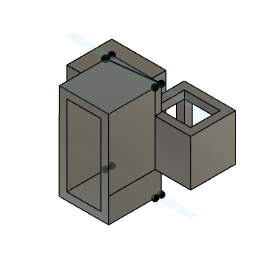
DrzacZaALUFrameKojiDrziKameruZaNogaruStola v4 (Autodesk Fusion 360 design; units mm, degrees)
Autodesk Fusion 360 part; units mm, degrees
sketch "Sketch1" plane through (0, 0, 0) normal (0, 0, 1) x (1, 0, 0)
  line L0 (100, 50) -> (100, 20)
  line L1 (100, 50) -> (150, 50)
  line L2 (120, 20) -> (100, 20)
  line L3 (70, 50) -> (70, 70)
  line L4 (70, 70) -> (150, 70)
  line L5 (100, 50) -> (120, 50)
  line L6 (120, 50) -> (120, 20)
  line L7 (150, 50) -> (150, 70)
  line L8 (150, 50) -> (100, 50)
  line L9 (70, 50) -> (150, 50)
  line L10 (120, 50) -> (150, 50)
  line L11 (100, 50) -> (70, 50)
  line L12 (120, 50) -> (125, 50)
  line L13 (125, 20) -> (125, 50)
  line L14 (125, 20) -> (120, 20)
  line L15 (100, 20) -> (95, 20)
  line L16 (95, 20) -> (95, 50)
  dimension "d1" = 30
  dimension "d2" = 50
  dimension "d3" = 20
  constraint horizontal L9
  constraint coincident L0.start L9
  constraint perpendicular L0 L1
  constraint perpendicular L0 L2
  constraint perpendicular L3 L9
  constraint perpendicular L0 L4
  constraint perpendicular L0 L5
  constraint perpendicular L2 L6
  constraint perpendicular L4 L7
  constraint midpoint L1 L12.end
  constraint perpendicular L8 L13
  constraint perpendicular L6 L14
  constraint perpendicular L0 L15
  constraint coincident L11 L16.end
  measures "d1" distance of L0.start L0.end
  measures "d2" distance of L0.start L1.end
  measures "d3" distance of L0.start L5.end
extrude "Extrude1" add sketch "Sketch1" along normal blind 60
sketch "Sketch2" plane through (0, 20, 0) normal (0, -1, 0) x (1, 0, 0)
  line L0 (95, 0) -> (125, 0)
  line L1 (125, 0) -> (125, 60)
  line L2 (125, 60) -> (95, 60)
  line L3 (95, 60) -> (95, 0)
  line L4 (95, 0) -> (100, 0)
  line L5 (100, 0) -> (100, 55)
  line L6 (100, 55) -> (120, 55)
  line L7 (120, 55) -> (120, 5)
  line L8 (120, 5) -> (100, 5)
  line L9 (-15, -85) -> (-10, -80)
  dimension "d6" = 5
  constraint coincident L0.start L3.end
  constraint perpendicular L3 L4
  constraint perpendicular L4 L5
  constraint perpendicular L5 L6
  constraint perpendicular L6 L7
  constraint coincident L5 L8.end
  constraint perpendicular L5 L8
  measures "d6" distance of L0.start L4.end
extrude "Extrude2" add 1 faces at (105, 63.3333, 60) along direction (0, 0, 1) blind 2
extrude "Extrude3" cut sketch "Sketch2" against normal blind 30 contours L5 L6 L7 L8
extrude "Extrude4" cut 1 faces at (106.6667, 30, 55) along direction (0, 0, 1) blind 2
extrude "Extrude5" add 1 faces at (125, 30, 20.6667) along direction (1, 0, 0) blind 2
extrude "Extrude6" cut 1 faces at (120, 30, 39.6667) along direction (1, 0, 0) blind 2
sketch "Sketch3" plane through (0, 70, 0) normal (0, 1, 0) x (-1, 0, 0)
  line L0 (-150, 0) -> (-70, 0)
  line L1 (-70, 0) -> (-70, 62)
  line L2 (-70, 62) -> (-150, 62)
  line L3 (-150, 62) -> (-150, 0)
  line L4 (-70, 31) -> (-150, 31)
  line L5 (-150, 31) -> (-150, 16)
  line L6 (-150, 31) -> (-150, 46)
  line L7 (-150, 16) -> (-70, 16)
  line L8 (-150, 46) -> (-70, 46)
  dimension "d17" = 15
  dimension "d18" = 15
  constraint midpoint L1 L4.start
  constraint midpoint L3 L4.end
  constraint perpendicular L4 L5
  constraint perpendicular L4 L6
  constraint coincident L1 L7.end
  constraint perpendicular L1 L7
  constraint coincident L1 L8.end
  constraint perpendicular L1 L8
  measures "d17" distance of L4.end L5.end
  measures "d18" distance of L4.end L6.end
extrude "Extrude7" cut sketch "Sketch3" against normal blind 16 contours L0 L1 L3 L7 | L1 L2 L3 L8
sketch "Sketch4" plane through (0, 0, 0) normal (0, 0, -1) x (1, 0, 0)
  line L0 (70, -54) -> (150, -54)
  line L1 (150, -54) -> (150, -50)
  line L2 (150, -50) -> (127, -50)
  line L3 (127, -50) -> (127, -20)
  line L4 (127, -20) -> (95, -20)
  line L5 (95, -20) -> (95, -50)
  line L6 (95, -50) -> (70, -50)
  line L7 (70, -50) -> (70, -54)
  line L8 (127, -50) -> (127, -54)
  line L9 (95, -50) -> (95, -54)
  constraint coincident L2.end L3.start
  constraint coincident L0 L8.end
  constraint perpendicular L0 L8
  constraint coincident L5.end L6.start
  constraint coincident L0 L9.end
  constraint perpendicular L0 L9
sketch "Sketch5" plane through (0, 54, 0) normal (0, 1, 0) x (-1, 0, 0)
  line L0 (-150, 0) -> (-70, 0)
  line L1 (-70, 0) -> (-70, 16)
  line L2 (-70, 16) -> (-150, 16)
  line L3 (-150, 16) -> (-150, 0)
  line L4 (-95, 0) -> (-95, 16)
  line L5 (-126.9826, 0) -> (-126.9826, 16)
  constraint coincident L0 L4.start
  constraint coincident L2 L4.end
  constraint perpendicular L2 L4
  constraint coincident L0 L5.start
  constraint coincident L2 L5.end
  constraint perpendicular L2 L5
extrude "Extrude8" cut sketch "Sketch5" against normal blind 50 contours L0 L2 L3 L5 | L0 L1 L2 L4
sketch "Sketch6" plane through (0, 0, 62) normal (0, 0, 1) x (-1, 0, 0)
  line L0 (-150, -54) -> (-70, -54)
  line L1 (-70, -54) -> (-70, -50)
  line L2 (-70, -50) -> (-95, -50)
  line L3 (-95, -50) -> (-95, -20)
  line L4 (-95, -20) -> (-127, -20)
  line L5 (-127, -20) -> (-127, -50)
  line L6 (-127, -50) -> (-150, -50)
  line L7 (-150, -50) -> (-150, -54)
  line L8 (-127, -50) -> (-127, -54)
  line L9 (-127, -54) -> (-95, -50)
  line L10 (-95, -54) -> (-95, -50)
  constraint coincident L5.end L6.start
  constraint coincident L0 L8.end
  constraint perpendicular L0 L8
  constraint coincident L2.end L3.start
  constraint coincident L0 L10.start
  constraint perpendicular L2 L10
sketch "Sketch7" plane through (0, 54, 0) normal (0, 1, 0) x (-1, 0, 0)
  line L0 (-150, 46) -> (-70, 46)
  line L1 (-70, 46) -> (-70, 62)
  line L2 (-70, 62) -> (-150, 62)
  line L3 (-150, 62) -> (-150, 46)
  line L4 (-95.1201, 62) -> (-95.1201, 46)
  line L5 (-127.0485, 62) -> (-127.0485, 46)
  constraint coincident L2 L4.start
  constraint coincident L0 L4.end
  constraint perpendicular L0 L4
  constraint coincident L2 L5.start
  constraint coincident L0 L5.end
  constraint perpendicular L0 L5
extrude "Extrude9" cut sketch "Sketch7" against normal blind 50 contours L0 L2 L3 L5 | L0 L1 L2 L4
sketch "Sketch8" plane through (0, 0, 0) normal (0, 0, -1) x (1, 0, 0)
extrude "Extrude10" add 1 faces at (96.6667, 70, 36) along direction (0, 1, 0) blind 9
sketch "Sketch9" plane through (0, 0, 62) normal (0, 0, 1) x (1, 0, 0)
sketch "Sketch10" plane through (70, 0, 0) normal (-1, 0, 0) x (0, -1, 0)
  line L0 (-50, 46) -> (-79, 46)
  line L1 (-79, 46) -> (-79, 16)
  line L2 (-79, 16) -> (-50, 16)
  line L3 (-50, 16) -> (-50, 46)
  line L4 (-74, 27.7711) -> (-74, 16)
  line L5 (-74, 27.7711) -> (-74, 46)
  line L6 (-74, 46) -> (-54, 46)
  line L7 (-54, 16) -> (-54, 46)
  line L8 (-54, 16) -> (-54, 21)
  line L9 (-54, 21) -> (-74, 21)
  line L10 (-74, 21) -> (-74, 41)
  line L11 (-74, 41) -> (-54, 41)
  dimension "d28" = 20
  dimension "d29" = 5
  dimension "d30" = 20
  constraint coincident L2 L4.end
  constraint perpendicular L2 L4
  constraint coincident L0 L5.end
  constraint perpendicular L0 L5
  constraint perpendicular L3 L6
  constraint coincident L2 L7.start
  constraint perpendicular L6 L7
  constraint perpendicular L2 L8
  constraint coincident L4 L9.end
  constraint perpendicular L4 L9
  constraint perpendicular L9 L10
  constraint coincident L7 L11.end
  constraint perpendicular L7 L11
  measures "d28" distance of L5.end L6.end
  measures "d29" distance of L7.start L8.end
  measures "d30" distance of L9.end L10.end
extrude "Extrude11" cut sketch "Sketch10" against normal blind 500 contours L4 L5 L7 L9 L10 L11
sketch "Sketch11" plane through (0, 0, 0) normal (0, 1, 0) x (1, 0, 0)
sketch "Sketch12" plane through (0, 79, 0) normal (0, 1, 0) x (-1, 0, 0)
  line L0 (-150, 16) -> (-70, 16)
  line L1 (-70, 16) -> (-70, 46)
  line L2 (-70, 46) -> (-150, 46)
  line L3 (-150, 46) -> (-150, 16)
  line L4 (-94.9405, 16) -> (-94.9405, 46)
  line L5 (-126.875, 16) -> (-126.875, 46)
  line L6 (-94.9405, 16) -> (-99.9405, 16)
  line L7 (-126.875, 16) -> (-121.875, 16)
  line L8 (-99.9405, 16) -> (-105, 16)
  line L9 (-121.875, 16) -> (-116.875, 16)
  line L10 (-105, 16) -> (-105, 46)
  line L11 (-116.875, 16) -> (-116.875, 46)
  dimension "d33" = 5
  dimension "d34" = 5
  dimension "d35" = 5
  constraint coincident L0 L4.start
  constraint coincident L2 L4.end
  constraint perpendicular L2 L4
  constraint coincident L0 L5.start
  constraint coincident L2 L5.end
  constraint perpendicular L2 L5
  constraint perpendicular L4 L6
  constraint perpendicular L5 L7
  constraint coincident L0 L8.end
  constraint parallel L0 L8
  constraint parallel L0 L9
  constraint coincident L2 L10.end
  constraint perpendicular L2 L10
  constraint coincident L2 L11.end
  constraint perpendicular L2 L11
  measures "d33" distance of L4.start L6.end
  measures "d34" distance of L5.start L7.end
  measures "d35" distance of L7.end L9.end
extrude "Extrude12" cut sketch "Sketch12" against normal blind 25 contours L0 L2 L10 L11
sketch "Sketch13" plane through (0, 79, 0) normal (0, 1, 0) x (-1, 0, 0)
  line L0 (-105, 46) -> (-105, 16)
  line L1 (-105, 16) -> (-70, 16)
  line L2 (-70, 16) -> (-70, 46)
  line L3 (-70, 46) -> (-105, 46)
  line L4 (-70, 16) -> (-75, 16)
  line L5 (-70, 16) -> (-70, 21)
  line L6 (-105, 46) -> (-105, 41)
  line L7 (-105, 46) -> (-100, 46)
  line L8 (-105, 16) -> (-105, 17)
  line L9 (-105, 16) -> (-105, 21)
  line L10 (-105, 16) -> (-100, 16)
  line L11 (-70, 46) -> (-75, 46)
  line L12 (-70, 46) -> (-70, 41)
  line L13 (-94, 41) -> (-81, 41)
  line L14 (-75, 25.1667) -> (-75, 36.8333)
  line L15 (-100, 25.1667) -> (-100, 36.8333)
  line L16 (-81, 21) -> (-94, 21)
  line L17 (-75, 36.8333) -> (-82, 31)
  line L18 (-87.5, 26.4167) -> (-94, 21)
  line L19 (-81, 41) -> (-87.5, 35.5833)
  line L20 (-93, 31) -> (-100, 25.1667)
  line L21 (-100, 36.8333) -> (-93, 31)
  line L22 (-87.5, 26.4167) -> (-81, 21)
  line L23 (-75, 25.1667) -> (-82, 31)
  line L24 (-87.5, 35.5833) -> (-94, 41)
  dimension "d38" = 5
  dimension "d39" = 5
  dimension "d40" = 5
  dimension "d41" = 5
  dimension "d42" = 5
  dimension "d43" = 5
  dimension "d44" = 5
  constraint coincident L1.end L2.start
  constraint coincident L0.start L3.end
  constraint coincident L1 L4.end
  constraint perpendicular L2 L4
  constraint perpendicular L4 L5
  constraint perpendicular L3 L6
  constraint perpendicular L6 L7
  constraint coincident L0.end L1.start
  constraint coincident L0 L8.end
  constraint perpendicular L1 L8
  constraint perpendicular L1 L9
  constraint perpendicular L8 L10
  constraint coincident L2.end L3.start
  constraint perpendicular L2 L11
  constraint perpendicular L11 L12
  constraint perpendicular L13 L14
  constraint perpendicular L13 L15
  constraint collinear L17 L18
  constraint coincident L19.end L23
  constraint collinear L19 L20
  constraint coincident L18.start L21
  constraint collinear L21 L22
  constraint collinear L23 L24
  measures "d38" distance of L1.end L5.end
  measures "d39" distance of L0.start L6.end
  measures "d40" distance of L0.start L7.end
  measures "d41" distance of L0.end L9.end
  measures "d42" distance of L0.end L10.end
  measures "d43" distance of L2.end L11.end
  measures "d44" distance of L2.end L12.end
extrude "Extrude13" cut sketch "Sketch13" against normal blind 5 contours L13 L19 L24 | L14 L17 L23 | L15 L20 L21 | L16 L18 L22
sketch "Sketch14" plane through (0, 79, 0) normal (0, 1, 0) x (-1, 0, 0)
  line L0 (-116.875, 16) -> (-116.875, 46)
  line L1 (-116.875, 46) -> (-150, 46)
  line L2 (-150, 46) -> (-150, 16)
  line L3 (-150, 16) -> (-116.875, 16)
sketch "Sketch15" plane through (0, 0, 46) normal (0, 0, 1) x (-1, 0, 0)
  line L0 (-105, -54) -> (-105, -79)
  line L1 (-105, -79) -> (-70, -79)
  line L2 (-70, -79) -> (-70, -50)
  line L3 (-70, -50) -> (-95, -50)
  line L4 (-95, -50) -> (-95, -20)
  line L5 (-95, -20) -> (-95.1201, -20)
  line L6 (-95.1201, -20) -> (-95.1201, -54)
  line L7 (-95.1201, -54) -> (-105, -54)
  line L8 (-84.9539, -79) -> (-84.9539, -74)
  line L9 (-84.9539, -74) -> (-84.9539, -64)
  circle A0 centre (-84.9539, -64) radius 2.5
  dimension "d47" = 5
  dimension "d48" = 10
  dimension "d49" = 5
  constraint coincident L1 L8.start
  constraint perpendicular L1 L8
  constraint parallel L8 L9
  constraint coincident L9.end A0.centre
  measures "d47" distance of L8.start L8.end
  measures "d48" distance of L8.end L9.end
  measures "d49" diameter of A0
extrude "Extrude14" cut sketch "Sketch15" against normal blind 10 contours A0
sketch "Sketch16" plane through (0, 79, 0) normal (0, 1, 0) x (-1, 0, 0)
  line L0 (-81, 21) -> (-94, 21)
  line L1 (-94, 21) -> (-87.5, 26.4167)
  line L2 (-87.5, 26.4167) -> (-81, 21)
  line L3 (-75, 25.1667) -> (-82, 31)
  line L4 (-82, 31) -> (-75, 36.8333)
  line L5 (-75, 36.8333) -> (-75, 25.1667)
  line L6 (-93, 31) -> (-100, 25.1667)
  line L7 (-100, 25.1667) -> (-100, 36.8333)
  line L8 (-100, 36.8333) -> (-93, 31)
  line L9 (-94, 41) -> (-81, 41)
  line L10 (-81, 41) -> (-87.5, 35.5833)
  line L11 (-87.5, 35.5833) -> (-94, 41)
  line L12 (-105, 46) -> (-105, 16)
  line L13 (-105, 16) -> (-70, 16)
  line L14 (-70, 16) -> (-70, 46)
  line L15 (-70, 46) -> (-105, 46)
  line L16 (-117, 16) -> (-122, 16)
  line L17 (-117, 16) -> (-117, 21)
  line L18 (-117, 46) -> (-122, 46)
  line L19 (-117, 46) -> (-117, 41)
  line L20 (-150, 46) -> (-145, 46)
  line L21 (-150, 46) -> (-150, 41)
  line L22 (-150, 16) -> (-145, 16)
  line L23 (-150, 16) -> (-150, 21)
  line L24 (-150, 21) -> (-117, 21)
  line L25 (-122, 16) -> (-122, 46)
  line L26 (-117, 41) -> (-150, 41)
  line L27 (-145, 46) -> (-145, 16)
  dimension "d52" = 5
  dimension "d53" = 5
  dimension "d54" = 5
  dimension "d55" = 5
  dimension "d56" = 5
  dimension "d57" = 5
  dimension "d58" = 5
  dimension "d59" = 5
  constraint horizontal L16
  constraint perpendicular L16 L17
  constraint horizontal L18
  constraint perpendicular L18 L19
  constraint horizontal L20
  constraint perpendicular L20 L21
  constraint horizontal L22
  constraint perpendicular L22 L23
  constraint perpendicular L17 L24
  constraint perpendicular L18 L25
  constraint perpendicular L21 L26
  constraint perpendicular L22 L27
  measures "d52" distance of L16.start L16.end
  measures "d53" distance of L16.start L17.end
  measures "d54" distance of L18.start L18.end
  measures "d55" distance of L18.start L19.end
  measures "d56" distance of L20.start L20.end
  measures "d57" distance of L20.start L21.end
  measures "d58" distance of L22.start L22.end
  measures "d59" distance of L22.start L23.end
extrude "Extrude15" cut sketch "Sketch16" against normal blind 6 contours L24 L25 L26 L27
sketch "Sketch17" plane through (0, 0, 46) normal (0, 0, 1) x (-1, 0, 0)
  circle A0 centre (-84.9539, -64) radius 2.5
  line L0 (-105, -54) -> (-105, -79)
  line L1 (-105, -79) -> (-70, -79)
  line L2 (-70, -79) -> (-70, -50)
  line L3 (-70, -50) -> (-95, -50)
  line L4 (-95, -50) -> (-95, -20)
  line L5 (-95, -20) -> (-95.1201, -20)
  line L6 (-95.1201, -20) -> (-95.1201, -54)
  line L7 (-95.1201, -54) -> (-105, -54)
  line L8 (-117, -79) -> (-122, -79)
  line L9 (-117, -79) -> (-117, -74)
  line L10 (-150, -79) -> (-150, -74)
  line L11 (-150, -79) -> (-145, -79)
  line L12 (-150, -50) -> (-150, -55)
  line L13 (-150, -50) -> (-145, -50)
  line L14 (-145, -50) -> (-117, -50)
  line L15 (-117, -50) -> (-117, -55)
  line L16 (-117, -55) -> (-117, -50)
  line L17 (-117, -50) -> (-122, -50)
  line L18 (-122, -79) -> (-122, -50)
  line L19 (-117, -55) -> (-150, -55)
  line L20 (-145, -50) -> (-145, -79)
  line L21 (-150, -74) -> (-117, -74)
  dimension "d62" = 5
  dimension "d63" = 5
  dimension "d64" = 5
  dimension "d65" = 5
  dimension "d66" = 5
  constraint horizontal L8
  constraint perpendicular L8 L9
  constraint vertical L10
  constraint perpendicular L10 L11
  constraint vertical L12
  constraint perpendicular L12 L13
  constraint perpendicular L12 L14
  constraint perpendicular L14 L15
  constraint perpendicular L16 L17
  constraint perpendicular L12 L19
  constraint parallel L18 L20
  constraint perpendicular L9 L21
  measures "d62" distance of L8.start L9.end
  measures "d63" distance of L10.start L10.end
  measures "d64" distance of L10.start L11.end
  measures "d65" distance of L12.start L12.end
  measures "d66" distance of L14.end L17.end
extrude "Extrude16" cut sketch "Sketch17" against normal blind 6 contours L18 L19 L20 L21
sketch "Sketch18" plane through (0, 0, 16) normal (0, 0, -1) x (1, 0, 0)
  line L0 (116.875, -54) -> (116.875, -79)
  line L1 (116.875, -79) -> (150, -79)
  line L2 (150, -79) -> (150, -50)
  line L3 (150, -50) -> (127, -50)
  line L4 (127, -50) -> (127, -20)
  line L5 (127, -20) -> (126.9826, -20)
  line L6 (126.9826, -20) -> (126.9826, -54)
  line L7 (126.9826, -54) -> (116.875, -54)
  line L8 (150, -79) -> (145, -79)
  line L9 (150, -79) -> (150, -75)
  line L10 (150, -50) -> (145, -50)
  line L11 (150, -50) -> (150, -55)
  line L12 (116.875, -79) -> (116.875, -74)
  line L13 (116.875, -79) -> (121.875, -79)
  line L14 (127, -50) -> (117, -50)
  line L15 (117, -50) -> (117, -58)
  line L16 (117, -58) -> (117, -50)
  line L17 (117, -50) -> (117, -55)
  line L18 (117, -50) -> (122, -50)
  line L19 (122, -50) -> (121.875, -79)
  line L20 (117, -55) -> (150, -55)
  line L21 (145, -50) -> (145, -79)
  line L22 (150, -75) -> (150, -74)
  line L23 (150, -74) -> (116.875, -74)
  dimension "d69" = 5
  dimension "d70" = 5
  dimension "d71" = 5
  dimension "d72" = 5
  dimension "d73" = 5
  dimension "d74" = 5
  dimension "d75" = 5
  dimension "d76" = 1
  constraint coincident L1.end L2.start
  constraint perpendicular L2 L8
  constraint coincident L2 L9.end
  constraint perpendicular L1 L9
  constraint coincident L2.end L3.start
  constraint perpendicular L2 L10
  constraint perpendicular L10 L11
  constraint coincident L0.end L1.start
  constraint perpendicular L1 L12
  constraint perpendicular L12 L13
  constraint coincident L3.end L4.start
  constraint perpendicular L4 L14
  constraint perpendicular L7 L15
  constraint perpendicular L7 L17
  constraint perpendicular L17 L18
  constraint parallel L2 L22
  measures "d69" distance of L1.end L8.end
  measures "d70" distance of L2.end L10.end
  measures "d71" distance of L2.end L11.end
  measures "d72" distance of L0.end L12.end
  measures "d73" distance of L0.end L13.end
  measures "d74" distance of L14.end L17.end
  measures "d75" distance of L14.end L18.end
  measures "d76" distance of L9.end L22.end
extrude "Extrude17" cut sketch "Sketch18" against normal blind 6 contours L19 L20 L21 L23
sketch "Sketch19" plane through (0, 0, 16) normal (0, 0, -1) x (1, 0, 0)
  line L0 (105, -79) -> (105, -54)
  line L1 (105, -54) -> (95, -54)
  line L2 (95, -54) -> (95, -50)
  line L3 (95, -50) -> (70, -50)
  line L4 (70, -50) -> (70, -79)
  line L5 (70, -79) -> (105, -79)
  line L6 (105, -79) -> (100, -79)
  line L7 (105, -79) -> (105, -74)
  line L8 (70, -79) -> (70, -74)
  line L9 (70, -79) -> (75, -79)
  line L10 (70, -50) -> (70, -55)
  line L11 (70, -50) -> (75, -50)
  line L12 (105, -54) -> (105, -50)
  line L13 (105, -50) -> (105, -55)
  line L14 (105, -50) -> (100, -50)
  line L15 (100, -50) -> (105, -50)
  line L16 (100, -79) -> (100, -50)
  line L17 (105, -55) -> (70, -55)
  line L18 (75, -50) -> (75, -79)
  line L19 (70, -74) -> (105, -74)
  dimension "d79" = 5
  dimension "d80" = 5
  dimension "d81" = 5
  dimension "d82" = 5
  dimension "d83" = 5
  dimension "d84" = 5
  dimension "d85" = 5
  dimension "d86" = 5
  constraint coincident L0.start L5.end
  constraint perpendicular L0 L6
  constraint perpendicular L6 L7
  constraint coincident L4.end L5.start
  constraint perpendicular L5 L8
  constraint perpendicular L8 L9
  constraint coincident L3.end L4.start
  constraint perpendicular L3 L10
  constraint perpendicular L4 L11
  constraint coincident L0.end L1.start
  constraint perpendicular L1 L12
  constraint perpendicular L1 L13
  constraint perpendicular L12 L14
  constraint perpendicular L12 L15
  measures "d79" distance of L0.start L6.end
  measures "d80" distance of L0.start L7.end
  measures "d81" distance of L4.end L8.end
  measures "d82" distance of L4.end L9.end
  measures "d83" distance of L3.end L10.end
  measures "d84" distance of L3.end L11.end
  measures "d85" distance of L12.end L13.end
  measures "d86" distance of L14.end L12.end
extrude "Extrude18" cut sketch "Sketch19" against normal blind 6 contours L16 L17 L18 L19
extrude "Extrude19" add 1 faces at (146.6667, 74, 34.3333) along direction (0, -1, 0) blind 20
